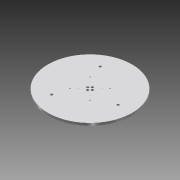
# Autodesk Inventor part: Base_Can
Saved by Autodesk Inventor 2014 (Build 180170000, 170)
## iProperties
Created: 2014-02-01
Part Number: Base_Can
Material: Generic
Document SubType Name: Modeling
Designer: Owner
Density: 1 g/cm^3
Appearance: Aluminum - Polished
Author: Owner
Autodesk Inventor part; units mm, degrees
ref_plane "YZ Plane" through (0, 0, 0) normal (1, 0, 0) x (0, 1, 0)
ref_plane "XZ Plane" through (0, 0, 0) normal (0, 1, 0) x (-1, 0, 0)
ref_plane "XY Plane" through (0, 0, 0) normal (0, 0, 1) x (1, 0, 0)
sketch "Sketch1" plane through (0, 0, 0) normal (0, 1, 0) x (-1, 0, 0)
  circle A0 centre (0, 0) radius 225.425
  dimension "d0" = 450.85
  constraints: 1 centre point, 1 coincident
  measures "d0" diameter of A0
extrude "Extrusion1" add sketch "Sketch1" along normal blind 12.7
sketch "Sketch2" plane through (0, 12.7, 0) normal (0, 1, 0) x (1, 0, 0)
  circle A0 centre (0, 0) radius 225.425 projected
  circle A1 centre (0, 12.7) radius 6.35
  dimension "d3" = 12.7
  dimension "d4" = 12.7
  constraints: 1 centre point
  measures "d3" diameter of A1
  measures "d4" distance of A0.centre A1.centre
extrude "Extrusion2" cut sketch "Sketch2" against normal blind 12.7 contours A1
pattern_circular "Circular Pattern1" count 4 over 360 about axis through (0, -10, 0) along (0, 1, 0) of "Extrusion2"
sketch "Sketch3" plane through (0, 12.7, 0) normal (0, 1, 0) x (1, 0, 0)
  circle A0 centre (0, 0) radius 225.425 projected
  line L0 (-38.1, 38.1) -> (38.1, 38.1)
  line L1 (38.1, 38.1) -> (38.1, -38.1)
  line L2 (38.1, -38.1) -> (-38.1, -38.1)
  line L3 (-38.1, -38.1) -> (-38.1, 38.1)
  circle A1 centre (-31.75, 31.75) radius 1.5875
  circle A2 centre (31.75, 31.75) radius 1.5875
  circle A3 centre (-31.75, -31.75) radius 1.5875
  circle A4 centre (31.75, -31.75) radius 1.5875
  line L4 (-63.5, 63.5) -> (63.5, 63.5)
  line L5 (63.5, 63.5) -> (63.5, -63.5)
  line L6 (63.5, -63.5) -> (-63.5, -63.5)
  line L7 (-63.5, -63.5) -> (-63.5, 63.5)
  circle A5 centre (53.975, 53.975) radius 3.175
  circle A6 centre (-53.975, 53.975) radius 3.175
  circle A7 centre (53.975, -53.975) radius 3.175
  circle A8 centre (-53.975, -53.975) radius 3.175
  circle A9 centre (150.495, 0) radius 6.35
  circle A10 centre (-75.2475, 130.3325) radius 6.35
  circle A11 centre (-75.2475, -130.3325) radius 6.35
  dimension "d10" = 76.2
  dimension "d11" = 76.2
  dimension "d12" = 38.1
  dimension "d13" = 38.1
  dimension "d14" = 3.175
  dimension "d15" = 6.35
  dimension "d16" = 6.35
  dimension "d19" = 63.5
  dimension "d22" = 63.5
  dimension "d27" = 127
  dimension "d28" = 127
  dimension "d29" = 63.5
  dimension "d30" = 63.5
  dimension "d31" = 6.35
  dimension "d32" = 9.525
  dimension "d33" = 9.525
  dimension "d36" = 107.95
  dimension "d39" = 107.95
  dimension "d42" = 12.7
  dimension "d43" = 150.495
  dimension "d46" = 360
  constraints: 16 end point, 11 centre point, 4 horizontal, 4 parallel, 2 perpendicular, 2 vertical, 19 other
  measures "d10" distance of L0.start L0.end
  measures "d11" distance of L0.end L1.end
  measures "d12" distance from line of A0.centre L0
  measures "d13" distance from line of L1 A0.centre
  measures "d14" diameter of A1
  measures "d15" distance from line of L0 A1.centre
  measures "d16" distance from line of L3 A1.centre
  measures "d19" distance of A1.centre A2.centre
  measures "d22" distance of A1.centre A3.centre
  measures "d27" distance of L4.start L4.end
  measures "d28" distance of L4.end L5.end
  measures "d29" distance from line of A0.centre L4
  measures "d30" distance from line of L5 A0.centre
  measures "d31" diameter of A5
  measures "d32" distance from line of L5 A5.centre
  measures "d33" distance from line of L4 A5.centre
  measures "d36" distance of A5.centre A6.centre
  measures "d39" distance of A5.centre A7.centre
  measures "d42" diameter of A9
  measures "d43" distance of A0.centre A9.centre
extrude "Extrusion3" cut sketch "Sketch3" against normal blind 12.7 contours A1 | A2 | A3 | A4 | A5 | A6 | A7 | A8 | A9 | A10 | A11
body "Solid1"
